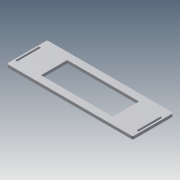
# Autodesk Inventor part: TopFrontPanel
Saved by Autodesk Inventor 2014 (Build 180170000, 170)
## iProperties
Created: 2014-08-11
Part Number: TopFrontPanel
Material: Generic
Document SubType Name: Modeling
Designer: Peele
Density: 1 g/cm^3
Appearance: White
Author: Peele
Autodesk Inventor part; units mm, degrees
ref_plane "YZ Plane" through (0, 0, 0) normal (1, 0, 0) x (0, 1, 0)
ref_plane "XZ Plane" through (0, 0, 0) normal (0, 1, 0) x (-1, 0, 0)
ref_plane "XY Plane" through (0, 0, 0) normal (0, 0, 1) x (1, 0, 0)
sketch "Sketch1" plane through (0, 0, 0) normal (0, 0, 1) x (1, 0, 0)
  line L0 (-132, -42.5) -> (132, -42.5)
  line L1 (132, -42.5) -> (132, 42.5)
  line L2 (132, 42.5) -> (-132, 42.5)
  line L3 (-132, 42.5) -> (-132, -42.5)
  line L4 (-132, -42.5) -> (132, 42.5) construction
  line L5 (132, -42.5) -> (-132, 42.5) construction
  point P0 (0, 0)
  dimension "d0" = 85
  dimension "d1" = 264
  constraints: 12 end point, 2 midpoint, 2 parallel, 1 horizontal, 1 perpendicular
  measures "d0" distance of L2.end L0.start
  measures "d1" distance of L0.start L0.end
extrude "Extrusion1" add sketch "Sketch1" along normal blind 6
sketch "Sketch2" plane through (0, 0, 6) normal (0, 0, 1) x (1, 0, 0)
  line L0 (-132, -42.5) -> (132, -42.5) projected
  line L1 (132, -42.5) -> (132, 42.5) projected
  line L2 (-129, -27.5) -> (-125, -27.5)
  line L3 (-125, -27.5) -> (-125, 22.5)
  line L4 (-125, 22.5) -> (-129, 22.5)
  line L5 (-129, 22.5) -> (-129, -27.5)
  line L6 (-129, -27.5) -> (-125, 22.5) construction
  line L7 (-125, -27.5) -> (-129, 22.5) construction
  line L8 (125, -27.5) -> (129, -27.5)
  line L9 (129, -27.5) -> (129, 22.5)
  line L10 (129, 22.5) -> (125, 22.5)
  line L11 (125, 22.5) -> (125, -27.5)
  line L12 (125, -27.5) -> (129, 22.5) construction
  line L13 (129, -27.5) -> (125, 22.5) construction
  point P0 (0, 0)
  point P1 (-127, -2.5)
  point P2 (127, -2.5)
  dimension "d4" = 258
  dimension "d5" = 3
  dimension "d6" = 4
  dimension "d7" = 50
  dimension "d8" = 15
  constraints: 24 end point, 4 midpoint, 4 parallel, 2 equal length, 2 horizontal, 2 perpendicular, 1 collinear
  measures "d4" distance between parallel lines of L9 L5
  measures "d5" distance between parallel lines of L9 L1
  measures "d6" distance of L9.end L10.end
  measures "d7" distance of L2.end L3.end
  measures "d8" distance between parallel lines of L2 L0
extrude "Extrusion2" cut sketch "Sketch2" against normal blind 4
fillet "Fillet1" radius 3 4 edges at (132, -42.5, 3) (132, 42.5, 3) (-132, -42.5, 3) (-132, 42.5, 3)
sketch "Sketch4" plane through (0, 0, 6) normal (0, 0, 1) x (1, 0, 0)
  line L0 (75, -27.5) -> (-75, -27.5)
  line L1 (-75, -27.5) -> (-75, 27.5)
  line L2 (-75, 27.5) -> (75, 27.5)
  line L3 (75, 27.5) -> (75, -27.5)
  line L4 (75, -27.5) -> (-75, 27.5) construction
  line L5 (-75, -27.5) -> (75, 27.5) construction
  line L6 (129, 42.5) -> (-129, 42.5) projected
  line L7 (-125, 22.5) -> (-125, -27.5) projected
  point P0 (0, 0)
  dimension "d32" = 50
  dimension "d33" = 15
  constraints: 12 end point, 2 midpoint, 2 parallel, 1 horizontal, 1 perpendicular
  measures "d32" distance between parallel lines of L7 L1
  measures "d33" distance between parallel lines of L6 L2
extrude "Extrusion5" cut sketch "Sketch4" against normal blind 10
body "Solid1"
